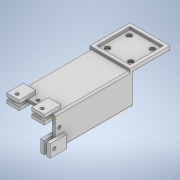
# Autodesk Inventor part: carriageEnd2R
Saved by Autodesk Inventor 2020 (Build 240168000, 168)
## iProperties
Created: 2020-01-10
Part Number: carriageEnd2R
Material: Generic
Document SubType Name: Modeling
Designer: PAB
Density: 1 g/cm^3
Appearance: Default
Author: PAB
Autodesk Inventor part; units mm, degrees
ref_plane "YZ Plane" through (0, 0, 0) normal (1, 0, 0) x (0, 1, 0)
ref_plane "XZ Plane" through (0, 0, 0) normal (0, 1, 0) x (-1, 0, 0)
ref_plane "XY Plane" through (0, 0, 0) normal (0, 0, 1) x (1, 0, 0)
sketch "Sketch1" plane through (0, 0, 0) normal (0, 1, 0) x (-1, 0, 0)
  line L0 (24, 138) -> (-24, 138)
  line L1 (-24, 138) -> (-24, -138)
  line L2 (-24, -138) -> (24, -138)
  line L3 (24, -138) -> (24, 138)
  point P0 (0, 0)
  dimension "d0" = 48
  dimension "d1" = 276
  constraints: 8 end point, 2 parallel, 1 horizontal, 1 perpendicular
  measures "d0" distance of L2.end L1.end
  measures "d1" distance of L1.end L0.end
extrude "Extrusion1" add sketch "Sketch1" along normal blind 3
sketch "Sketch2" plane through (0, 3, 0) normal (0, 1, 0) x (1, 0, 0)
  line L0 (-24, 138) -> (-24, -138) projected
  line L1 (-24, -138) -> (-20, -138)
  line L2 (-20, -138) -> (-20, -90)
  line L3 (-20, -90) -> (-24, -90)
  line L4 (-24, -90) -> (-24, -138)
  line L5 (24, -138) -> (24, 138) projected
  line L6 (-20, -90) -> (24, -90)
  line L7 (24, -90) -> (24, -94)
  line L8 (24, -94) -> (-20, -94)
  line L9 (-20, -94) -> (-20, -90)
  line L10 (-24, -138) -> (24, -138) projected
  line L11 (24, -94) -> (20, -94)
  line L12 (20, -94) -> (20, -138)
  line L13 (20, -138) -> (24, -138)
  line L14 (24, -138) -> (24, -94)
  line L15 (20, -138) -> (-20, -138)
  line L16 (-20, -138) -> (-20, -134)
  line L17 (-20, -134) -> (20, -134)
  line L18 (20, -134) -> (20, -138)
  point P0 (0, 0)
  dimension "d4" = 4
  dimension "d5" = 48
  dimension "d6" = 4
  dimension "d7" = 4
  dimension "d8" = 4
  constraints: 32 end point, 8 parallel, 4 horizontal, 4 perpendicular, 3 point on line
  measures "d4" distance of L3.end L2.end
  measures "d5" distance of L2.end L1.end
  measures "d6" distance of L6.end L7.end
  measures "d7" distance of L13.end L12.end
  measures "d8" distance of L15.end L16.end
extrude "Extrusion2" add sketch "Sketch2" along normal blind 3 contours L3 L2 L1 L0 | L6 L5 L8 L2 | L2 L17 L12 L10 | L12 L8 L5 L10
mirror "Mirror1" about plane through (0, 0, 0) normal (0, 0, 1) of "Extrusion2"
sketch "Sketch3" plane through (0, 0, 0) normal (0, -1, 0) x (1, 0, 0)
  line L0 (24, -90) -> (-24, -90) projected
  line L1 (24, 138) -> (24, -138) projected
  line L2 (-24, -90) -> (24, -90)
  line L3 (24, -90) -> (24, -93)
  line L4 (24, -93) -> (-24, -93)
  line L5 (-24, -93) -> (-24, -90)
  line L6 (-24, 90) -> (24, 90) projected
  line L7 (24, 90) -> (21, 90)
  line L8 (21, 90) -> (21, -90)
  line L9 (21, -90) -> (24, -90)
  line L10 (24, -90) -> (24, 90)
  line L11 (-24, 90) -> (24, 90)
  line L12 (24, 90) -> (24, 93)
  line L13 (24, 93) -> (-24, 93)
  line L14 (-24, 93) -> (-24, 90)
  point P0 (0, 0)
  dimension "d11" = 3
  dimension "d12" = 3
  dimension "d13" = 3
  constraints: 24 end point, 6 parallel, 3 horizontal, 3 perpendicular, 3 point on line
  measures "d11" distance of L2.end L3.end
  measures "d12" distance of L9.end L8.end
  measures "d13" distance of L12.end L11.end
extrude "Extrusion3" add sketch "Sketch3" along normal blind 35
sketch "Sketch4" plane through (-24, 0, -90) normal (0, 0, 1) x (1, 0, 0)
  line L0 (0, -35) -> (45, -35) projected
  line L1 (45, 0) -> (45, -35) projected
  line L2 (0, -35) -> (45, -35)
  line L3 (45, -35) -> (45, -31)
  line L4 (45, -31) -> (0, -31)
  line L5 (0, -31) -> (0, -35)
  point P0 (24, 0)
  dimension "d16" = 4
  constraints: 8 end point, 2 parallel, 1 horizontal, 1 perpendicular, 1 point on line
  measures "d16" distance of L3.end L2.end
extrude "Extrusion4" add sketch "Sketch4" along normal blind 8
sketch "Sketch5" plane through (-24, -31, -90) normal (0, 1, 0) x (1, 0, 0)
  line L0 (0, -8) -> (45, -8) projected
  line L1 (45, 0) -> (45, -8) projected
  line L2 (0, -8) -> (45, -8)
  line L3 (45, -8) -> (45, -4)
  line L4 (45, -4) -> (0, -4)
  line L5 (0, -4) -> (0, -8)
  point P0 (24, -90)
  dimension "d19" = 4
  constraints: 8 end point, 2 parallel, 1 horizontal, 1 midpoint, 1 perpendicular
  measures "d19" distance of L3.end L2.end
extrude "Extrusion5" add sketch "Sketch5" along normal blind 4
sketch "Sketch6" plane through (0, 0, 0) normal (0, -1, 0) x (1, 0, 0)
  line L0 (21, -86) -> (-24, -86) projected
  line L1 (-24, -82) -> (21, -82)
  line L2 (21, -82) -> (21, -86)
  line L3 (21, -86) -> (-24, -86)
  line L4 (-24, -86) -> (-24, -82)
  point P0 (0, 0)
  dimension "d22" = 4
  constraints: 8 end point, 2 parallel, 1 horizontal, 1 perpendicular
  measures "d22" distance of L1.end L0.start
extrude "Extrusion6" add sketch "Sketch6" along normal blind 4
mirror "Mirror2" about plane through (0, 0, 0) normal (0, 0, 1) of "Extrusion6", "Extrusion5", "Extrusion4"
sketch "Sketch7" plane through (0, 0, 0) normal (0, -1, 0) x (1, 0, 0)
  circle A0 centre (-14, -127) radius 3
  circle A1 centre (14, -127) radius 3
  circle A2 centre (14, -101) radius 3
  circle A3 centre (-14, -101) radius 3
  line L0 (-20, -94) -> (20, -94) projected
  line L1 (20, -134) -> (-20, -134) projected
  line L2 (20, -94) -> (20, -134) projected
  point P0 (0, 0)
  dimension "d25" = 6
  dimension "d26" = 6
  dimension "d27" = 6
  dimension "d28" = 6
  dimension "d80" = 28
  dimension "d81" = 26
  dimension "d82" = 26
  dimension "d83" = 28
  dimension "d84" = 7
  dimension "d85" = 7
  dimension "d86" = 7
  dimension "d87" = 6
  constraints: 4 centre point
  measures "d25" diameter of A0
  measures "d26" diameter of A1
  measures "d27" diameter of A2
  measures "d28" diameter of A3
  measures "d80" distance of A2.centre A3.centre
  measures "d81" distance of A3.centre A0.centre
  measures "d82" distance of A2.centre A1.centre
  measures "d83" distance of A1.centre A0.centre
  measures "d84" distance from line of L0 A2.centre
  measures "d85" distance from line of L0 A3.centre
  measures "d86" distance from line of L1 A0.centre
  measures "d87" distance from line of L2 A2.centre
extrude "Extrusion7" cut sketch "Sketch7" against normal blind 4
mirror "Mirror3" about plane through (0, 0, 0) normal (0, 0, 1) of "Extrusion7"
sketch "Sketch12" plane through (0, 0, 0) normal (0, -1, 0) x (1, 0, 0)
  line L0 (-24, -82) -> (-24, 82) projected
  line L1 (-24, 0) -> (24, 0)
  line L2 (24, 0) -> (24, 138)
  line L3 (24, 138) -> (-24, 138)
  line L4 (-24, 138) -> (-24, 0)
  point P0 (0, 0)
  point P1 (-24, -17)
  constraints: 8 end point, 2 parallel, 1 horizontal, 1 midpoint, 1 perpendicular
extrude "Extrusion12" cut sketch "Sketch12" along normal mid plane 100
sketch "Sketch13" plane through (0, 0, 0) normal (0, -1, 0) x (1, 0, 0)
  line L0 (-24, -90) -> (-24, 0) projected
  line L1 (-24, -10) -> (-9, -10)
  line L2 (-9, -10) -> (-9, 10)
  line L3 (-9, 10) -> (-24, 10)
  line L4 (-24, 10) -> (-24, -10)
  line L5 (6, -10) -> (21, -10)
  line L6 (21, -10) -> (21, 10)
  line L7 (21, 10) -> (6, 10)
  line L8 (6, 10) -> (6, -10)
  point P0 (0, 0)
  dimension "d55" = 15
  dimension "d56" = 20
  dimension "d57" = 15
  dimension "d58" = 20
  constraints: 16 end point, 4 parallel, 2 horizontal, 2 perpendicular, 2 point on line
  measures "d55" distance of L3.end L2.end
  measures "d56" distance of L2.end L1.end
  measures "d57" distance of L7.end L6.end
  measures "d58" distance of L6.end L5.end
extrude "Extrusion13" add sketch "Sketch13" along normal blind 4 and the other way blind 7
sketch "Sketch14" plane through (21, -31, -90) normal (-1, 0, 0) x (0, 0, 1)
  point P0 (90, 31)
sketch "Sketch15" plane through (21, -31, -90) normal (-1, 0, 0) x (0, 0, 1)
  line L0 (90, -4) -> (8, -4) projected
  line L1 (80, -4) -> (100, -4)
  line L2 (100, -4) -> (100, 11)
  line L3 (100, 11) -> (80, 11)
  line L4 (80, 11) -> (80, -4)
  point P0 (90, 31)
  dimension "d63" = 20
  dimension "d64" = 15
  constraints: 8 end point, 2 parallel, 1 horizontal, 1 perpendicular, 1 point on line
  measures "d63" distance of L3.end L2.end
  measures "d64" distance of L2.end L1.end
extrude "Extrusion14" add sketch "Sketch15" along normal blind 4 and the other way blind 7
sketch "Sketch16" plane through (0, -4, 0) normal (0, -1, 0) x (1, 0, 0)
  circle A0 centre (-16.5, 5) radius 2
  circle A1 centre (13.5, 5) radius 2
  circle A2 centre (-1.5, -5) radius 2
  point P0 (0, 0)
  dimension "d69" = 4
  dimension "d70" = 4
  dimension "d71" = 4
  constraints: 3 centre point
  measures "d69" diameter of A0
  measures "d70" diameter of A1
  measures "d71" diameter of A2
extrude "Extrusion15" cut sketch "Sketch16" against normal blind 20
sketch "Sketch17" plane through (17, -31, -90) normal (-1, 0, 0) x (0, 0, 1)
  circle A0 centre (95, 3.5) radius 2
  circle A1 centre (85, 18.5) radius 2
  point P0 (90, 31)
  dimension "d74" = 4
  dimension "d75" = 4
  constraints: 2 centre point
  measures "d74" diameter of A0
  measures "d75" diameter of A1
extrude "Extrusion16" cut sketch "Sketch17" against normal blind 20
sketch "Sketch18" plane through (-24, -4, 10) normal (0, 0, 1) x (1, 0, 0)
  line L0 (48, 4) -> (48, -31) projected
  line L1 (45, -31) -> (45, -16) projected
  line L2 (48, -31) -> (45, -31)
  line L3 (45, -31) -> (45, -16)
  line L4 (45, -16) -> (48, -16)
  line L5 (48, -16) -> (48, -31)
  line L6 (48, 7) -> (0, 7) projected
  line L7 (45, 4) -> (0, 4)
  line L8 (0, 4) -> (0, 7)
  line L9 (0, 7) -> (45, 7)
  line L10 (45, 7) -> (45, 4)
  point P0 (24, 4)
  constraints: 16 end point, 4 parallel, 2 horizontal, 2 perpendicular
extrude "Extrusion17" cut sketch "Sketch18" against normal blind 10
fillet "Fillet1" radius 2 7 edges at (24, -35, -51.5) (24, 3, -45) (-24, 3, -50) (-24, 0, -115.5) (0, 0, -138) (24, 0, -115.5) (0, -35, -93)
body "Solid1"
